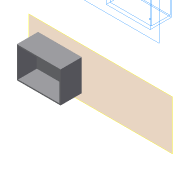
# Autodesk Inventor part: 10_MiniSPIM_Samplechamber
Saved by Autodesk Inventor 2019 (Build 230136000, 136)
## iProperties
Created: 2019-10-13
Part Number: 10_MiniSPIM_Samplechamber
Material: Generic
Document SubType Name: Modeling
Designer: diederichbenedict
Density: 1 g/cm^3
Appearance: Default
Author: diederichbenedict
Autodesk Inventor part; units mm, degrees
ref_plane "YZ Plane" through (0, 0, 0) normal (1, 0, 0) x (0, 1, 0)
ref_plane "XZ Plane" through (0, 0, 0) normal (0, 1, 0) x (-1, 0, 0)
ref_plane "XY Plane" through (0, 0, 0) normal (0, 0, 1) x (1, 0, 0)
ref_plane "Work Plane1" through (0, 0, 0) normal (0, 0, 1) x (1, 0, 0)
sketch "Sketch1" plane through (0, 0, 0) normal (0, 0, 1) x (1, 0, 0)
  arc A0 (-74.415, -11.0527) -> (-74.415, -5.9883) centre (-76.6839, -8.5205) ccw projected
  line L0 (-74.415, -11.3137) -> (-74.415, -11.0527) projected
  line L1 (30, -11.3137) -> (-74.415, -11.3137) projected
  line L2 (30, 11.3137) -> (30, -11.3137) projected
  line L3 (25, 11.3137) -> (30, 11.3137) projected
  line L4 (0, 11.3137) -> (25, 11.3137) projected
  line L5 (-25, 11.3137) -> (0, 11.3137) projected
  line L6 (-30, 11.3137) -> (-25, 11.3137) projected
  line L7 (-30, 16.3137) -> (-30, 11.3137) projected
  line L8 (-30, 24.6863) -> (-30, 16.3137) projected
  line L9 (-74.415, 24.6863) -> (-30, 24.6863) projected
  line L10 (-74.415, -5.9883) -> (-74.415, 24.6863) projected
  line L11 (-72.2851, 17.6802) -> (-37.2851, 17.6802)
  line L12 (-37.2851, 17.6802) -> (-37.2851, -7.3198)
  line L13 (-37.2851, -7.3198) -> (-72.2851, -7.3198)
  line L14 (-72.2851, -7.3198) -> (-72.2851, 17.6802)
  point P0 (0, 0)
  dimension "d0" = 35
  dimension "d1" = 25
  constraints: 8 end point, 2 parallel, 1 horizontal, 1 perpendicular
  measures "d0" distance of L12.end L13.end
  measures "d1" distance of L11.end L12.end
extrude "Extrusion1" add sketch "Sketch1" along normal blind 2 contours L11 L12 L13 L14
sketch "Sketch2" plane through (0, 0, 2) normal (0, 0, 1) x (1, 0, 0)
  line L0 (-37.2851, 17.6802) -> (-72.2851, 17.6802) projected
  line L1 (-72.2851, 17.6802) -> (-72.2851, -7.3198) projected
  line L2 (-72.2851, -7.3198) -> (-37.2851, -7.3198) projected
  line L3 (-37.2851, -7.3198) -> (-37.2851, 17.6802) projected
  line L4 (-38.2851, 16.6802) -> (-71.2851, 16.6802)
  line L5 (-71.2851, 16.6802) -> (-71.2851, -6.3198)
  line L6 (-71.2851, -6.3198) -> (-38.2851, -6.3198)
  line L7 (-38.2851, -6.3198) -> (-38.2851, 16.6802)
  point P0 (0, 0)
  dimension "d4" = 1
  constraints: 8 end point, 3 other
  measures "d4" distance between parallel lines of L3 L7
extrude "Extrusion2" add sketch "Sketch2" along normal blind 18
sketch "Sketch3" plane through (-72.2851, -7.3198, 0) normal (-1, 0, 0) x (0, 0, 1)
  line L0 (0, 0) -> (0, 25) projected
  line L1 (0, 0) -> (20, 0) projected
  line L2 (20, 25) -> (20, 0) projected
  line L3 (0, 25) -> (20, 25) projected
  line L4 (2.5, 23.088) -> (14.5, 23.088)
  line L5 (14.5, 23.088) -> (14.5, 11.088)
  line L6 (14.5, 11.088) -> (2.5, 11.088)
  line L7 (2.5, 11.088) -> (2.5, 23.088)
  line L8 (2.5, 23.088) -> (14.5, 11.088) construction
  line L9 (14.5, 23.088) -> (2.5, 11.088) construction
  point P0 (0, 7.3198)
  point P1 (8.5, 17.088)
  dimension "d7" = 12
  dimension "d8" = 12
  constraints: 12 end point, 2 midpoint, 2 parallel, 1 horizontal, 1 perpendicular
  measures "d7" distance of L5.end L6.end
  measures "d8" distance of L4.end L5.end
extrude "Extrusion3" cut sketch "Sketch3" against normal blind 15 contours L4 L5 L6 L7
sketch "Sketch4" plane through (-72.2851, 17.6802, 0) normal (0, 1, 0) x (1, 0, 0)
  line L0 (0, 0) -> (35, 0) projected
  line L1 (0, 0) -> (0, -20) projected
  line L2 (35, -20) -> (0, -20) projected
  line L3 (35, 0) -> (35, -20) projected
  line L4 (17.4558, -2.5) -> (5.4558, -2.5)
  line L5 (5.4558, -2.5) -> (5.4558, -14.5)
  line L6 (5.4558, -14.5) -> (17.4558, -14.5)
  line L7 (17.4558, -14.5) -> (17.4558, -2.5)
  line L8 (17.4558, -2.5) -> (5.4558, -14.5) construction
  line L9 (5.4558, -2.5) -> (17.4558, -14.5) construction
  point P0 (72.2851, 0)
  point P1 (11.4558, -8.5)
  dimension "d11" = 12
  dimension "d12" = 12
  constraints: 12 end point, 2 midpoint, 2 parallel, 1 horizontal, 1 perpendicular
  measures "d11" distance of L6.end L5.end
  measures "d12" distance of L5.end L4.end
extrude "Extrusion4" cut sketch "Sketch4" against normal through all contours L7 L6 L5 L4
body "Solid1"
